rob3_v2 (Autodesk Fusion 360 design; units mm, degrees)
Autodesk Fusion 360 part; units mm, degrees
sketch "Sketch1" plane through (0, 0, 0) normal (0, 0, 1) x (1, 0, 0)
  spline S0 degree 5 poles (0, 0.083) (3.4028, 0.6487) (10.1655, 1.6592) (20.1813, 2.8133) (33.3011, 3.6916) (49.3449, 3.7981) (61.865, 3.0163) (71.0307, 1.8175) (77.0289, 0.7123) (80, 0.083) knots 0 0 0 0 0 0 0.2 0.4 0.6 0.8 1 1 1 1 1 1
  line L0 (72.4946, 1.6726) -> (87.5054, -1.5065)
  line L1 (-8.6308, -1.3517) -> (8.6308, 1.5177)
  spline S1 degree 5 poles (0, 17.083) (3.4028, 16.5174) (10.1655, 15.5068) (20.1813, 14.3528) (33.3011, 13.4745) (49.3449, 13.368) (61.865, 14.1497) (71.0307, 15.3485) (77.0289, 16.4538) (80, 17.083) knots 0 0 0 0 0 0 0.2 0.4 0.6 0.8 1 1 1 1 1 1
  line L2 (-8.6308, 18.5177) -> (8.6308, 15.6483)
  line L3 (72.4946, 15.4935) -> (87.5054, 18.6726)
  line L4 (80, 17.083) -> (80, 0.083)
  line L5 (0, 17.083) -> (0, 0.083)
  circle A0 centre (40, 8.5) radius 2.6
  dimension "d13" = 5.2
  dimension "d14" = 40
  dimension "d15" = 40
  dimension "d18" = 17
  dimension "d21" = 17
  dimension "d22" = 8.5
  constraint midpoint S0.end L0
  constraint midpoint L1 S0.start
  constraint vertical L4
  constraint vertical L5
  measures "d13" diameter of A0
  measures "d14" distance of S1.start A0.centre
  measures "d15" distance of S1.end A0.centre
  measures "d18" distance of S0.end S1.end
  measures "d21" distance of S0.start S1.start
  measures "d22" vertical distance of origin A0.centre
extrude "Extrude4" add sketch "Sketch1" along normal blind 4
extrude "Extrude2" [suppressed]
extrude "Extrude3" [suppressed]
equation "d22 = ( 17 / 2 ) * 1 mm"
